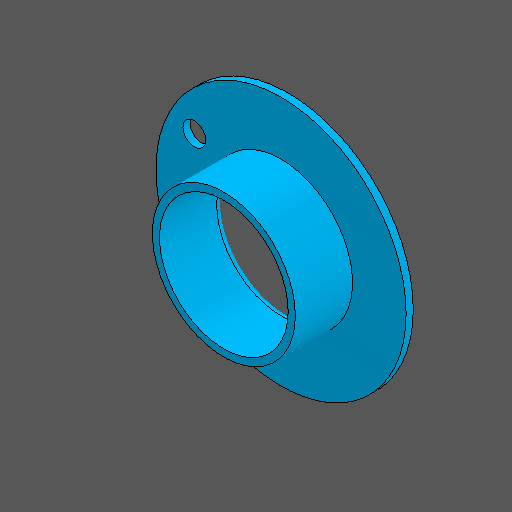
# Autodesk Inventor part: Pre-Anode
Saved by Autodesk Inventor 2025 (Build 290162000, 162)
## iProperties
Created: 2024-05-16
Part Number: Pre-Anode
Material: Stainless Steel
Document SubType Name: Modeling
Designer: KAA
Density: 8 g/cm^3
Appearance: Sky Blue Medium
Mass: 9.41699 g
Surface Area: 25.308 cm^2
Volume: 1.17712 cm^3
Author: KAA
Autodesk Inventor part; units mm, degrees
ref_plane "YZ Plane" through (0, 0, 0) normal (1, 0, 0) x (0, 1, 0)
ref_plane "XZ Plane" through (0, 0, 0) normal (0, 1, 0) x (-1, 0, 0)
ref_plane "XY Plane" through (0, 0, 0) normal (0, 0, 1) x (1, 0, 0)
sketch "Sketch1" plane through (0, 0, 0) normal (0, 0, 1) x (1, 0, 0)
  circle A0 centre (0, 0) radius 10
  circle A1 centre (0, 0) radius 17.5
  dimension "d0" = 35
  dimension "d1" = 20
  constraints: 2 centre point, 2 coincident
  measures "d0" diameter of A1
  measures "d1" diameter of A0
extrude "Extrusion1" add sketch "Sketch1" along normal blind 1
sketch "Sketch2" plane through (0, 0, 1) normal (0, 0, 1) x (1, 0, 0)
  circle A0 centre (-12.1244, 7) radius 1.6
  circle A1 centre (0, 0) radius 10 projected
  circle A2 centre (0, 0) radius 17.5 projected
  line L0 (0, 0) -> (-10, 0) construction
  line L1 (-15.1554, 8.75) -> (-8.6603, 5) construction
  circle A3 centre (0, 0) radius 14 construction
  point P0 (-11.9078, 6.875)
  dimension "d16" = 28
  dimension "d4" = 3.2
  dimension "d8" = 30
  constraints: 4 end point, 2 point on circle, 2 point on line, 1 centre point, 1 coincident, 1 horizontal, 1 midpoint, 5 other
  measures "d4" diameter of A0
  measures "d8" angle of L0 L1
extrude "Extrusion2" cut sketch "Sketch2" against normal through all contours A0
sketch "Sketch3" plane through (0, 0, 1) normal (0, 0, 1) x (1, 0, 0)
  circle A0 centre (0, 0) radius 9
  circle A1 centre (0, 0) radius 10
  circle A2 centre (0, 0) radius 10 projected
  dimension "d10" = 1
  dimension "d11" = 20
  constraints: 2 centre point, 2 coincident
  measures "d10" radial gap between concentric circles of A0 A1
  measures "d11" diameter of A1
extrude "Extrusion3" add sketch "Sketch3" along normal blind 8
sketch "Sketch4" plane through (0, 0, 1) normal (0, 0, -1) x (-1, 0, 0)
  circle A0 centre (0, 0) radius 9 projected
  circle A1 centre (0, 0) radius 10 projected
extrude "Extrusion4" add sketch "Sketch4" along normal up to surface (1 mm away)
fillet "Fillet1" radius 1 1 edges at (9, 0, 0)
body "Solid1"
